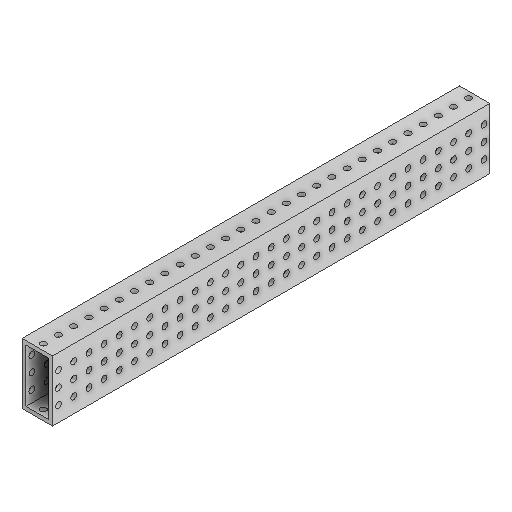
# Autodesk Inventor part: Foja - Base Chassi
Saved by Autodesk Inventor 2025.3 (Build 293356000, 356)
## iProperties
Created: 2026-05-13
Part Number: Foja - Base Chassi
Material: Genérico
Document SubType Name: Modeling
Designer: djair.oliveira
Density: 1 g/cm^3
Appearance: Padrão
Author: djair.oliveira
Autodesk Inventor part; units mm, degrees
ref_plane "YZ Plane" through (0, 0, 0) normal (1, 0, 0) x (0, 1, 0)
ref_plane "XZ Plane" through (0, 0, 0) normal (0, 1, 0) x (-1, 0, 0)
ref_plane "XY Plane" through (0, 0, 0) normal (0, 0, 1) x (1, 0, 0)
sketch "Esboço1" plane through (0, 0, 0) normal (0, 0, 1) x (1, 0, 0)
  line L0 (12.7, -25.4) -> (-12.7, -25.4)
  line L1 (-12.7, -25.4) -> (-12.7, 25.4)
  line L2 (-12.7, 25.4) -> (12.7, 25.4)
  line L3 (12.7, 25.4) -> (12.7, -25.4)
  line L4 (12.7, -25.4) -> (-12.7, 25.4) construction
  line L5 (-12.7, -25.4) -> (12.7, 25.4) construction
  line L6 (9.525, -22.225) -> (-9.525, -22.225)
  line L7 (-9.525, -22.225) -> (-9.525, 22.225)
  line L8 (-9.525, 22.225) -> (9.525, 22.225)
  line L9 (9.525, 22.225) -> (9.525, -22.225)
  line L10 (9.525, -22.225) -> (-9.525, 22.225) construction
  line L11 (-9.525, -22.225) -> (9.525, 22.225) construction
  point P0 (0, 0)
  dimension "d1" = 3.175
  dimension "d2" = 3.175
  dimension "d3" = 25.4
  dimension "d4" = 50.8
  constraints: 24 end point, 4 midpoint, 4 parallel, 2 horizontal, 2 perpendicular
  measures "d1" distance between parallel lines of L1 L7
  measures "d2" distance between parallel lines of L2 L8
  measures "d3" distance of L1.end L2.end
  measures "d4" distance of L2.end L0.start
extrude "Extrusão1" add sketch "Esboço1" along normal blind 386.4
sketch "Esboço2" plane through (-12.7, 25.4, 0) normal (0, 1, 0) x (1, 0, 0)
  circle A0 centre (12.7, -193.2) radius 2.5
  line L0 (0, 0) -> (0, -386.4) projected
  line L1 (25.4, -386.4) -> (0, -386.4) projected
  line L2 (25.4, 0) -> (0, 0) projected
  circle A1 centre (12.7, -205.9) radius 2.5
  circle A2 centre (12.7, -180.5) radius 2.5
  circle A3 centre (12.7, -218.6) radius 2.5
  circle A4 centre (12.7, -167.8) radius 2.5
  circle A5 centre (12.7, -231.3) radius 2.5
  circle A6 centre (12.7, -155.1) radius 2.5
  circle A7 centre (12.7, -244) radius 2.5
  circle A8 centre (12.7, -142.4) radius 2.5
  circle A9 centre (12.7, -256.7) radius 2.5
  circle A10 centre (12.7, -129.7) radius 2.5
  circle A11 centre (12.7, -269.4) radius 2.5
  circle A12 centre (12.7, -117) radius 2.5
  circle A13 centre (12.7, -282.1) radius 2.5
  circle A14 centre (12.7, -104.3) radius 2.5
  circle A15 centre (12.7, -294.8) radius 2.5
  circle A16 centre (12.7, -91.6) radius 2.5
  circle A17 centre (12.7, -307.5) radius 2.5
  circle A18 centre (12.7, -78.9) radius 2.5
  circle A19 centre (12.7, -320.2) radius 2.5
  circle A20 centre (12.7, -66.2) radius 2.5
  circle A21 centre (12.7, -332.9) radius 2.5
  circle A22 centre (12.7, -53.5) radius 2.5
  circle A23 centre (12.7, -345.6) radius 2.5
  circle A24 centre (12.7, -40.8) radius 2.5
  circle A25 centre (12.7, -358.3) radius 2.5
  circle A26 centre (12.7, -28.1) radius 2.5
  circle A27 centre (12.7, -371) radius 2.5
  circle A28 centre (12.7, -15.4) radius 2.5
  circle A29 centre (12.7, -383.7) radius 2.5
  circle A30 centre (12.7, -2.7) radius 2.5
  point P0 (12.7, 0)
  point P1 (12.7, -386.4)
  point P2 (12.7, 0)
  point P3 (12.7, 0)
  dimension "d7" = 5
  dimension "d8" = 12.7
  dimension "d9" = 386.4
  dimension "d10" = 193.2
  dimension "d13" = 12.7
  constraints: 31 centre point, 3 midpoint, 1 vertical, 60 other
  measures "d7" diameter of A0
  measures "d8" distance from line of L0 A0.centre
  measures "d9" distance of point (12.7, -386.4) point (12.7, 0)
  measures "d10" distance of point (12.7, 0) A0.centre
  measures "d13" distance of A0.centre A1.centre
extrude "Extrusão2" cut sketch "Esboço2" against normal up to surface (50.8 mm away)
sketch "Esboço3" plane through (12.7, -25.4, 0) normal (1, 0, 0) x (0, 0, -1)
  circle A0 centre (-193.2, 38.1) radius 2.5
  circle A1 centre (-193.2, 25.4) radius 2.5
  circle A2 centre (-193.2, 12.7) radius 2.5
  line L0 (0, 50.8) -> (-386.4, 50.8) projected
  line L1 (-193.2, 50.8) -> (-193.2, 0)
  line L2 (0, 0) -> (-386.4, 0) projected
  circle A3 centre (-205.9, 38.1) radius 2.5
  circle A4 centre (-205.9, 25.4) radius 2.5
  circle A5 centre (-205.9, 12.7) radius 2.5
  circle A6 centre (-180.5, 38.1) radius 2.5
  circle A7 centre (-180.5, 25.4) radius 2.5
  circle A8 centre (-180.5, 12.7) radius 2.5
  circle A9 centre (-218.6, 38.1) radius 2.5
  circle A10 centre (-218.6, 25.4) radius 2.5
  circle A11 centre (-218.6, 12.7) radius 2.5
  circle A12 centre (-167.8, 38.1) radius 2.5
  circle A13 centre (-167.8, 25.4) radius 2.5
  circle A14 centre (-167.8, 12.7) radius 2.5
  circle A15 centre (-231.3, 38.1) radius 2.5
  circle A16 centre (-231.3, 25.4) radius 2.5
  circle A17 centre (-231.3, 12.7) radius 2.5
  circle A18 centre (-155.1, 38.1) radius 2.5
  circle A19 centre (-155.1, 25.4) radius 2.5
  circle A20 centre (-155.1, 12.7) radius 2.5
  circle A21 centre (-244, 38.1) radius 2.5
  circle A22 centre (-244, 25.4) radius 2.5
  circle A23 centre (-244, 12.7) radius 2.5
  circle A24 centre (-142.4, 38.1) radius 2.5
  circle A25 centre (-142.4, 25.4) radius 2.5
  circle A26 centre (-142.4, 12.7) radius 2.5
  circle A27 centre (-256.7, 38.1) radius 2.5
  circle A28 centre (-256.7, 25.4) radius 2.5
  circle A29 centre (-256.7, 12.7) radius 2.5
  circle A30 centre (-129.7, 38.1) radius 2.5
  circle A31 centre (-129.7, 25.4) radius 2.5
  circle A32 centre (-129.7, 12.7) radius 2.5
  circle A33 centre (-269.4, 38.1) radius 2.5
  circle A34 centre (-269.4, 25.4) radius 2.5
  circle A35 centre (-269.4, 12.7) radius 2.5
  circle A36 centre (-117, 38.1) radius 2.5
  circle A37 centre (-117, 25.4) radius 2.5
  circle A38 centre (-117, 12.7) radius 2.5
  circle A39 centre (-282.1, 38.1) radius 2.5
  circle A40 centre (-282.1, 25.4) radius 2.5
  circle A41 centre (-282.1, 12.7) radius 2.5
  circle A42 centre (-104.3, 38.1) radius 2.5
  circle A43 centre (-104.3, 25.4) radius 2.5
  circle A44 centre (-104.3, 12.7) radius 2.5
  circle A45 centre (-294.8, 38.1) radius 2.5
  circle A46 centre (-294.8, 25.4) radius 2.5
  circle A47 centre (-294.8, 12.7) radius 2.5
  circle A48 centre (-91.6, 38.1) radius 2.5
  circle A49 centre (-91.6, 25.4) radius 2.5
  circle A50 centre (-91.6, 12.7) radius 2.5
  circle A51 centre (-307.5, 38.1) radius 2.5
  circle A52 centre (-307.5, 25.4) radius 2.5
  circle A53 centre (-307.5, 12.7) radius 2.5
  circle A54 centre (-78.9, 38.1) radius 2.5
  circle A55 centre (-78.9, 25.4) radius 2.5
  circle A56 centre (-78.9, 12.7) radius 2.5
  circle A57 centre (-320.2, 38.1) radius 2.5
  circle A58 centre (-320.2, 25.4) radius 2.5
  circle A59 centre (-320.2, 12.7) radius 2.5
  circle A60 centre (-66.2, 38.1) radius 2.5
  circle A61 centre (-66.2, 25.4) radius 2.5
  circle A62 centre (-66.2, 12.7) radius 2.5
  circle A63 centre (-332.9, 38.1) radius 2.5
  circle A64 centre (-332.9, 25.4) radius 2.5
  circle A65 centre (-332.9, 12.7) radius 2.5
  circle A66 centre (-53.5, 38.1) radius 2.5
  circle A67 centre (-53.5, 25.4) radius 2.5
  circle A68 centre (-53.5, 12.7) radius 2.5
  circle A69 centre (-345.6, 38.1) radius 2.5
  circle A70 centre (-345.6, 25.4) radius 2.5
  circle A71 centre (-345.6, 12.7) radius 2.5
  circle A72 centre (-40.8, 38.1) radius 2.5
  circle A73 centre (-40.8, 25.4) radius 2.5
  circle A74 centre (-40.8, 12.7) radius 2.5
  circle A75 centre (-358.3, 38.1) radius 2.5
  circle A76 centre (-358.3, 25.4) radius 2.5
  circle A77 centre (-358.3, 12.7) radius 2.5
  circle A78 centre (-28.1, 38.1) radius 2.5
  circle A79 centre (-28.1, 25.4) radius 2.5
  circle A80 centre (-28.1, 12.7) radius 2.5
  circle A81 centre (-371, 38.1) radius 2.5
  circle A82 centre (-371, 25.4) radius 2.5
  circle A83 centre (-371, 12.7) radius 2.5
  circle A84 centre (-15.4, 38.1) radius 2.5
  circle A85 centre (-15.4, 25.4) radius 2.5
  circle A86 centre (-15.4, 12.7) radius 2.5
  circle A87 centre (-383.7, 38.1) radius 2.5
  circle A88 centre (-383.7, 25.4) radius 2.5
  circle A89 centre (-383.7, 12.7) radius 2.5
  circle A90 centre (-2.7, 38.1) radius 2.5
  circle A91 centre (-2.7, 25.4) radius 2.5
  circle A92 centre (-2.7, 12.7) radius 2.5
  point P0 (0, 25.4)
  dimension "d20" = 5
  dimension "d21" = 25.4
  dimension "d22" = 12.7
  dimension "d23" = 12.7
  dimension "d26" = 12.7
  constraints: 93 centre point, 2 end point, 2 equal radius, 2 midpoint, 2 vertical alignment, 1 horizontal, 1 point on line, 180 other
  measures "d20" diameter of A1
  measures "d21" distance from line of L0 A1.centre
  measures "d22" distance of A0.centre A1.centre
  measures "d23" distance of A2.centre A1.centre
  measures "d26" distance of A0.centre A3.centre
extrude "Extrusão3" cut sketch "Esboço3" against normal up to surface (25.4 mm away)
sketch "Esboço4" plane through (-12.7, 25.4, 0) normal (0, 1, 0) x (1, 0, 0)
  circle A0 centre (12.7, -2.7) radius 2.5 projected
  circle A1 centre (12.7, -371) radius 2.5 projected
  circle A2 centre (12.7, -358.3) radius 2.5 projected
  circle A3 centre (12.7, -282.1) radius 2.5 projected
  circle A4 centre (12.7, -91.6) radius 2.5 projected
  circle A5 centre (12.7, -104.3) radius 2.5 projected
  circle A6 centre (12.7, -78.9) radius 2.5 projected
  circle A7 centre (12.7, -167.8) radius 2.5 projected
  circle A8 centre (12.7, -205.9) radius 2.5 projected
  circle A9 centre (12.7, -193.2) radius 2.5 projected
  circle A10 centre (12.7, -218.6) radius 2.5 projected
  circle A11 centre (12.7, -155.1) radius 2.5 projected
  circle A12 centre (12.7, -53.5) radius 2.5 projected
  circle A13 centre (12.7, -244) radius 2.5 projected
  circle A14 centre (12.7, -269.4) radius 2.5 projected
  circle A15 centre (12.7, -345.6) radius 2.5 projected
  circle A16 centre (12.7, -383.7) radius 2.5 projected
  circle A17 centre (12.7, -15.4) radius 2.5 projected
  circle A18 centre (12.7, -332.9) radius 2.5 projected
  circle A19 centre (12.7, -320.2) radius 2.5 projected
  circle A20 centre (12.7, -117) radius 2.5 projected
  circle A21 centre (12.7, -142.4) radius 2.5 projected
  circle A22 centre (12.7, -231.3) radius 2.5 projected
  circle A23 centre (12.7, -40.8) radius 2.5 projected
  circle A24 centre (12.7, -256.7) radius 2.5 projected
  circle A25 centre (12.7, -180.5) radius 2.5 projected
  circle A26 centre (12.7, -66.2) radius 2.5 projected
  circle A27 centre (12.7, -129.7) radius 2.5 projected
  circle A28 centre (12.7, -28.1) radius 2.5 projected
  circle A29 centre (12.7, -294.8) radius 2.5 projected
  circle A30 centre (12.7, -307.5) radius 2.5 projected
  line L0 (25.4, 0) -> (0, 0) projected
  line L1 (0, 0) -> (0, -386.4) projected
  line L2 (25.4, -386.4) -> (0, -386.4) projected
  line L3 (25.4, 0) -> (25.4, -386.4) projected
  line L4 (25.4, -376) -> (0, -376)
  line L5 (0, -10.4) -> (25.4, -10.4)
  point P0 (12.7, 0)
  dimension "d33" = 5
  dimension "d34" = 5
  constraints: 4 end point, 4 point on line, 1 horizontal, 1 perpendicular
  measures "d33" distance from line of A1.centre L4
  measures "d34" distance from line of A17.centre L5
extrude "Extrusão4" cut sketch "Esboço4" against normal up to surface (50.8 mm away) contours L3 L5 L1 L0 | L3 L2 L1 L4
equation "\"d2\" = d1"
equation "\"d10\" = 0.5 * d9"
equation "\"d23\" = d22"
